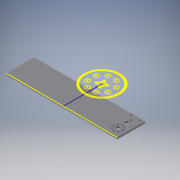
# Autodesk Inventor part: Winch Upright
Saved by Autodesk Inventor 2016 (Build 200138000, 138)
## iProperties
Created: 2015-12-16
Part Number: Winch Upright
Material: Generic
Document SubType Name: Modeling
Designer: Julia
Density: 1 g/cm^3
Appearance: Default
Author: Julia
Autodesk Inventor part; units mm, degrees
ref_plane "YZ Plane" through (0, 0, 0) normal (1, 0, 0) x (0, 1, 0)
ref_plane "XZ Plane" through (0, 0, 0) normal (0, 1, 0) x (-1, 0, 0)
ref_plane "XY Plane" through (0, 0, 0) normal (0, 0, 1) x (1, 0, 0)
sketch "Sketch1" plane through (0, 0, 0) normal (0, 1, 0) x (-1, 0, 0)
  line L0 (0, 0) -> (0, -50.8)
  line L1 (0, -50.8) -> (203.2, -50.8)
  line L2 (203.2, -50.8) -> (203.2, 0)
  line L3 (203.2, 0) -> (0, 0)
  dimension "d0" = 50.8
  dimension "d1" = 203.2
  constraints: 8 end point, 2 perpendicular, 1 horizontal, 1 vertical
  measures "d0" distance of L0.start L0.end
  measures "d1" distance of L0.end L1.end
extrude "Extrusion1" add sketch "Sketch1" along normal blind 3.302
sketch "Sketch2" plane through (0, 0, 0) normal (0, -1, 0) x (1, 0, 0)
  line L0 (-0.5, 0) -> (-0.5, -416) projected
  line L1 (-27.5, -416) -> (-0.5, -416) projected
  arc A0 (-30, -413.5) -> (-27.5, -416) centre (-27.5, -413.5) ccw projected
  line L2 (-30, -413.5) -> (-30, -2.5) projected
  arc A1 (-27.5, 0) -> (-30, -2.5) centre (-27.5, -2.5) ccw projected
  line L3 (-27.5, 0) -> (-0.5, 0) projected
  circle A2 centre (-14, -288) radius 4 projected
  circle A3 centre (-14, -320) radius 4 projected
  circle A4 centre (-14, -352) radius 4 projected
  circle A5 centre (-14, -384) radius 4 projected
  circle A6 centre (-14, -16) radius 4 projected
  circle A7 centre (-22, -16) radius 1.85 projected
  circle A8 centre (-6, -16) radius 1.85 projected
  circle A9 centre (-14, -24) radius 1.85 projected
  circle A10 centre (-14, -8) radius 1.85 projected
  circle A11 centre (-19.6569, -21.6569) radius 1.85 projected
  circle A12 centre (-19.6569, -10.3431) radius 1.85 projected
  circle A13 centre (-8.3431, -10.3431) radius 1.85 projected
  circle A14 centre (-8.3431, -21.6569) radius 1.85 projected
  circle A15 centre (-14, -80) radius 4 projected
  circle A16 centre (-22, -80) radius 1.85 projected
  circle A17 centre (-6, -80) radius 1.85 projected
  circle A18 centre (-14, -88) radius 1.85 projected
  circle A19 centre (-14, -72) radius 1.85 projected
  circle A20 centre (-19.6569, -85.6569) radius 1.85 projected
  circle A21 centre (-19.6569, -74.3431) radius 1.85 projected
  circle A22 centre (-8.3431, -74.3431) radius 1.85 projected
  circle A23 centre (-8.3431, -85.6569) radius 1.85 projected
  circle A24 centre (-14, -144) radius 4 projected
  circle A25 centre (-22, -144) radius 1.85 projected
  circle A26 centre (-6, -144) radius 1.85 projected
  circle A27 centre (-14, -152) radius 1.85 projected
  circle A28 centre (-14, -136) radius 1.85 projected
  circle A29 centre (-19.6569, -149.6569) radius 1.85 projected
  circle A30 centre (-19.6569, -138.3431) radius 1.85 projected
  circle A31 centre (-8.3431, -138.3431) radius 1.85 projected
  circle A32 centre (-8.3431, -149.6569) radius 1.85 projected
  circle A33 centre (-14, -208) radius 4 projected
  circle A34 centre (-22, -208) radius 1.85 projected
  circle A35 centre (-6, -208) radius 1.85 projected
  circle A36 centre (-14, -216) radius 1.85 projected
  circle A37 centre (-14, -200) radius 1.85 projected
  circle A38 centre (-19.6569, -213.6569) radius 1.85 projected
  circle A39 centre (-19.6569, -202.3431) radius 1.85 projected
  circle A40 centre (-8.3431, -202.3431) radius 1.85 projected
  circle A41 centre (-8.3431, -213.6569) radius 1.85 projected
  circle A42 centre (-14, -272) radius 4 projected
  circle A43 centre (-22, -272) radius 1.85 projected
  circle A44 centre (-6, -272) radius 1.85 projected
  circle A45 centre (-14, -280) radius 1.85 projected
  circle A46 centre (-14, -264) radius 1.85 projected
  circle A47 centre (-19.6569, -277.6569) radius 1.85 projected
  circle A48 centre (-19.6569, -266.3431) radius 1.85 projected
  circle A49 centre (-8.3431, -266.3431) radius 1.85 projected
  circle A50 centre (-8.3431, -277.6569) radius 1.85 projected
  circle A51 centre (-14, -336) radius 4 projected
  circle A52 centre (-22, -336) radius 1.85 projected
  circle A53 centre (-6, -336) radius 1.85 projected
  circle A54 centre (-14, -344) radius 1.85 projected
  circle A55 centre (-14, -328) radius 1.85 projected
  circle A56 centre (-19.6569, -341.6569) radius 1.85 projected
  circle A57 centre (-19.6569, -330.3431) radius 1.85 projected
  circle A58 centre (-8.3431, -330.3431) radius 1.85 projected
  circle A59 centre (-8.3431, -341.6569) radius 1.85 projected
  circle A60 centre (-14, -400) radius 4 projected
  circle A61 centre (-22, -400) radius 1.85 projected
  circle A62 centre (-6, -400) radius 1.85 projected
  circle A63 centre (-14, -408) radius 1.85 projected
  circle A64 centre (-14, -392) radius 1.85 projected
  circle A65 centre (-19.6569, -405.6569) radius 1.85 projected
  circle A66 centre (-19.6569, -394.3431) radius 1.85 projected
  circle A67 centre (-8.3431, -394.3431) radius 1.85 projected
  circle A68 centre (-8.3431, -405.6569) radius 1.85 projected
  circle A69 centre (-14, -48) radius 4 projected
  circle A70 centre (-22, -48) radius 1.85 projected
  circle A71 centre (-14, -56) radius 1.85 projected
  circle A72 centre (-6, -48) radius 1.85 projected
  circle A73 centre (-14, -40) radius 1.85 projected
  circle A74 centre (-14, -112) radius 4 projected
  circle A75 centre (-22, -112) radius 1.85 projected
  circle A76 centre (-14, -120) radius 1.85 projected
  circle A77 centre (-6, -112) radius 1.85 projected
  circle A78 centre (-14, -104) radius 1.85 projected
  circle A79 centre (-14, -176) radius 4 projected
  circle A80 centre (-22, -176) radius 1.85 projected
  circle A81 centre (-14, -184) radius 1.85 projected
  circle A82 centre (-6, -176) radius 1.85 projected
  circle A83 centre (-14, -168) radius 1.85 projected
  circle A84 centre (-14, -240) radius 4 projected
  circle A85 centre (-22, -240) radius 1.85 projected
  circle A86 centre (-14, -248) radius 1.85 projected
  circle A87 centre (-6, -240) radius 1.85 projected
  circle A88 centre (-14, -232) radius 1.85 projected
  circle A89 centre (-14, -304) radius 4 projected
  circle A90 centre (-22, -304) radius 1.85 projected
  circle A91 centre (-14, -312) radius 1.85 projected
  circle A92 centre (-6, -304) radius 1.85 projected
  circle A93 centre (-14, -296) radius 1.85 projected
  circle A94 centre (-14, -368) radius 4 projected
  circle A95 centre (-22, -368) radius 1.85 projected
  circle A96 centre (-14, -376) radius 1.85 projected
  circle A97 centre (-6, -368) radius 1.85 projected
  circle A98 centre (-14, -360) radius 1.85 projected
  circle A99 centre (-14, -32) radius 4 projected
  circle A100 centre (-14, -64) radius 4 projected
  circle A101 centre (-14, -96) radius 4 projected
  circle A102 centre (-14, -128) radius 4 projected
  circle A103 centre (-14, -160) radius 4 projected
  circle A104 centre (-14, -192) radius 4 projected
  circle A105 centre (-14, -224) radius 4 projected
  circle A106 centre (-14, -256) radius 4 projected
  point P0 (0, 0)
extrude "Extrusion2" cut sketch "Sketch2" against normal blind 20.5105 contours A6 | A7 | A8 | A9 | A10 | A11 | A12 | A13 | A14 | A70 | A72 | A73 | A99
sketch "Sketch3" plane through (0, 3.302, 0) normal (0, 1, 0) x (1, 0, 0)
  circle A0 centre (-98.9805, 70.6479) radius 6 projected
  arc A1 (-126.4697, 56.3203) -> (-127.7519, 54.8984) centre (-117.6318, 47.0611) ccw projected
  arc A2 (-127.7519, 54.8984) -> (-127.494, 54.4363) centre (-98.9805, 70.6479) ccw projected
  arc A3 (-127.494, 54.4363) -> (-125.6107, 54.7807) centre (-128.8482, 67.1645) ccw projected
  arc A4 (-125.6107, 54.7807) -> (-125.2608, 54.2076) centre (-98.9805, 70.6479) ccw projected
  arc A5 (-125.2608, 54.2076) -> (-126.4275, 52.6896) centre (-115.7237, 45.6704) ccw projected
  arc A6 (-126.4275, 52.6896) -> (-126.1342, 52.2491) centre (-98.9805, 70.6479) ccw projected
  arc A7 (-126.1342, 52.2491) -> (-124.2837, 52.7402) centre (-128.4828, 64.8318) ccw projected
  arc A8 (-124.2837, 52.7402) -> (-123.8899, 52.1964) centre (-98.9805, 70.6479) ccw projected
  arc A9 (-123.8899, 52.1964) -> (-124.9339, 50.5915) centre (-113.7124, 44.4337) ccw projected
  arc A10 (-124.9339, 50.5915) -> (-124.6069, 50.1754) centre (-98.9805, 70.6479) ccw projected
  arc A11 (-124.6069, 50.1754) -> (-122.8006, 50.8101) centre (-127.9355, 62.535) ccw projected
  arc A12 (-122.8006, 50.8101) -> (-122.3654, 50.2989) centre (-98.9805, 70.6479) ccw projected
  arc A13 (-122.3654, 50.2989) -> (-123.2803, 48.6171) centre (-111.6103, 43.3587) ccw projected
  arc A14 (-123.2803, 48.6171) -> (-122.9217, 48.2279) centre (-98.9805, 70.6479) ccw projected
  arc A15 (-122.9217, 48.2279) -> (-121.1708, 49.0024) centre (-127.2098, 60.2882) ccw projected
  arc A16 (-121.1708, 49.0024) -> (-120.6968, 48.5269) centre (-98.9805, 70.6479) ccw projected
  arc A17 (-120.6968, 48.5269) -> (-121.4768, 46.7784) centre (-109.4302, 42.4519) ccw projected
  arc A18 (-121.4768, 46.7784) -> (-121.0888, 46.4186) centre (-98.9805, 70.6479) ccw projected
  arc A19 (-121.0888, 46.4186) -> (-119.4041, 47.3281) centre (-126.3099, 58.1053) ccw projected
  arc A20 (-119.4041, 47.3281) -> (-118.8942, 46.8912) centre (-98.9805, 70.6479) ccw projected
  arc A21 (-118.8942, 46.8912) -> (-119.5347, 45.087) centre (-107.1858, 41.7189) ccw projected
  arc A22 (-119.5347, 45.087) -> (-119.1197, 44.7587) centre (-98.9805, 70.6479) ccw projected
  arc A23 (-119.1197, 44.7587) -> (-117.5114, 45.7976) centre (-125.2416, 55.9998) ccw projected
  arc A24 (-117.5114, 45.7976) -> (-116.9689, 45.4021) centre (-98.9805, 70.6479) ccw projected
  arc A25 (-116.9689, 45.4021) -> (-117.4659, 43.5531) centre (-104.8907, 41.1643) ccw projected
  arc A26 (-117.4659, 43.5531) -> (-117.0263, 43.2584) centre (-98.9805, 70.6479) ccw projected
  arc A27 (-117.0263, 43.2584) -> (-115.5046, 44.4202) centre (-124.0114, 53.9845) ccw projected
  arc A28 (-115.5046, 44.4202) -> (-114.9327, 44.0685) centre (-98.9805, 70.6479) ccw projected
  arc A29 (-114.9327, 44.0685) -> (-115.283, 42.1863) centre (-102.5593, 40.7915) ccw projected
  arc A30 (-115.283, 42.1863) -> (-114.8217, 41.927) centre (-98.9805, 70.6479) ccw projected
  arc A31 (-114.8217, 41.927) -> (-113.3958, 43.2046) centre (-122.6268, 52.072) ccw projected
  arc A32 (-113.3958, 43.2046) -> (-112.7981, 42.8989) centre (-98.9805, 70.6479) ccw projected
  arc A33 (-112.7981, 42.8989) -> (-112.9997, 40.9949) centre (-100.2057, 40.6028) ccw projected
  arc A34 (-112.9997, 40.9949) -> (-112.5195, 40.7726) centre (-98.9805, 70.6479) ccw projected
  arc A35 (-112.5195, 40.7726) -> (-111.1982, 42.1582) centre (-121.0964, 50.274) ccw projected
  arc A36 (-111.1982, 42.1582) -> (-110.5783, 41.9003) centre (-98.9805, 70.6479) ccw projected
  arc A37 (-110.5783, 41.9003) -> (-110.6299, 39.9864) centre (-97.8446, 40.5992) ccw projected
  arc A38 (-110.6299, 39.9864) -> (-110.1337, 39.8024) centre (-98.9805, 70.6479) ccw projected
  arc A39 (-110.1337, 39.8024) -> (-108.9253, 41.2874) centre (-119.4297, 48.6016) ccw projected
  arc A40 (-108.9253, 41.2874) -> (-108.2871, 41.0789) centre (-98.9805, 70.6479) ccw projected
  arc A41 (-108.2871, 41.0789) -> (-108.1884, 39.1669) centre (-95.4905, 40.781) ccw projected
  arc A42 (-108.1884, 39.1669) -> (-107.6793, 39.0225) centre (-98.9805, 70.6479) ccw projected
  arc A43 (-107.6793, 39.0225) -> (-106.591, 40.5977) centre (-117.637, 47.0651) ccw projected
  arc A44 (-106.591, 40.5977) -> (-105.9384, 40.4399) centre (-98.9805, 70.6479) ccw projected
  arc A45 (-105.9384, 40.4399) -> (-105.69, 38.5415) centre (-93.158, 41.1469) ccw projected
  arc A46 (-105.69, 38.5415) -> (-105.1711, 38.4375) centre (-98.9805, 70.6479) ccw projected
  arc A47 (-105.1711, 38.4375) -> (-104.2099, 40.0932) centre (-115.7292, 45.674) ccw projected
  arc A48 (-104.2099, 40.0932) -> (-103.5469, 39.9871) centre (-98.9805, 70.6479) ccw projected
  arc A49 (-103.5469, 39.9871) -> (-103.1503, 38.1141) centre (-90.8613, 41.6947) ccw projected
  arc A50 (-103.1503, 38.1141) -> (-102.6248, 38.051) centre (-98.9805, 70.6479) ccw projected
  arc A51 (-102.6248, 38.051) -> (-101.7964, 39.7771) centre (-113.7181, 44.4369) ccw projected
  arc A52 (-101.7964, 39.7771) -> (-101.1272, 39.7234) centre (-98.9805, 70.6479) ccw projected
  arc A53 (-101.1272, 39.7234) -> (-100.5848, 37.8872) centre (-88.6147, 42.4209) ccw projected
  arc A54 (-100.5848, 37.8872) -> (-100.0561, 37.8656) centre (-98.9805, 70.6479) ccw projected
  arc A55 (-100.0561, 37.8656) -> (-99.3657, 39.6513) centre (-111.6162, 43.3614) ccw projected
  arc A56 (-99.3657, 39.6513) -> (-98.6942, 39.6503) centre (-98.9805, 70.6479) ccw projected
  arc A57 (-98.6942, 39.6503) -> (-98.0095, 37.8623) centre (-86.4319, 43.3212) ccw projected
  arc A58 (-98.0095, 37.8623) -> (-97.4807, 37.8823) centre (-98.9805, 70.6479) ccw projected
  arc A59 (-97.4807, 37.8823) -> (-96.9325, 39.7167) centre (-109.4364, 42.4542) ccw projected
  arc A60 (-96.9325, 39.7167) -> (-96.2631, 39.7683) centre (-98.9805, 70.6479) ccw projected
  arc A61 (-96.2631, 39.7683) -> (-95.4402, 38.0396) centre (-84.3266, 44.39) ccw projected
  arc A62 (-95.4402, 38.0396) -> (-94.9146, 38.1009) centre (-98.9805, 70.6479) ccw projected
  arc A63 (-94.9146, 38.1009) -> (-94.512, 39.9727) centre (-107.1921, 41.7207) ccw projected
  arc A64 (-94.512, 39.9727) -> (-93.8487, 40.0767) centre (-98.9805, 70.6479) ccw projected
  arc A65 (-93.8487, 40.0767) -> (-92.8927, 38.4179) centre (-82.3116, 45.6207) ccw projected
  arc A66 (-92.8927, 38.4179) -> (-92.3735, 38.5203) centre (-98.9805, 70.6479) ccw projected
  arc A67 (-92.3735, 38.5203) -> (-92.119, 40.4179) centre (-104.8971, 41.1656) ccw projected
  arc A68 (-92.119, 40.4179) -> (-91.4659, 40.5736) centre (-98.9805, 70.6479) ccw projected
  arc A69 (-91.4659, 40.5736) -> (-90.3827, 38.9949) centre (-80.3994, 47.0057) ccw projected
  arc A70 (-90.3827, 38.9949) -> (-89.8731, 39.1377) centre (-98.9805, 70.6479) ccw projected
  arc A71 (-89.8731, 39.1377) -> (-89.7683, 41.0494) centre (-102.5657, 40.7923) ccw projected
  arc A72 (-89.7683, 41.0494) -> (-89.1294, 41.2559) centre (-98.9805, 70.6479) ccw projected
  arc A73 (-89.1294, 41.2559) -> (-87.9257, 39.767) centre (-78.6017, 48.5364) ccw projected
  arc A74 (-87.9257, 39.767) -> (-87.4289, 39.9494) centre (-98.9805, 70.6479) ccw projected
  arc A75 (-87.4289, 39.9494) -> (-87.4745, 41.8634) centre (-100.2122, 40.603) ccw projected
  arc A76 (-87.4745, 41.8634) -> (-86.8537, 42.1194) centre (-98.9805, 70.6479) ccw projected
  arc A77 (-86.8537, 42.1194) -> (-85.5369, 40.7296) centre (-76.9297, 50.2035) ccw projected
  arc A78 (-85.5369, 40.7296) -> (-85.056, 40.9503) centre (-98.9805, 70.6479) ccw projected
  arc A79 (-85.056, 40.9503) -> (-85.2515, 42.8549) centre (-97.8512, 40.599) ccw projected
  arc A80 (-85.2515, 42.8549) -> (-84.6528, 43.1588) centre (-98.9805, 70.6479) ccw projected
  arc A81 (-84.6528, 43.1588) -> (-83.231, 41.8765) centre (-75.3936, 51.9966) ccw projected
  arc A82 (-83.231, 41.8765) -> (-82.7689, 42.1344) centre (-98.9805, 70.6479) ccw projected
  arc A83 (-82.7689, 42.1344) -> (-83.1132, 44.0177) centre (-95.497, 40.7802) ccw projected
  arc A84 (-83.1132, 44.0177) -> (-82.5402, 44.3676) centre (-98.9805, 70.6479) ccw projected
  arc A85 (-82.5402, 44.3676) -> (-81.0222, 43.2009) centre (-74.0029, 53.9047) ccw projected
  arc A86 (-81.0222, 43.2009) -> (-80.5817, 43.4942) centre (-98.9805, 70.6479) ccw projected
  arc A87 (-80.5817, 43.4942) -> (-81.0727, 45.3448) centre (-93.1644, 41.1456) ccw projected
  arc A88 (-81.0727, 45.3448) -> (-80.5289, 45.7385) centre (-98.9805, 70.6479) ccw projected
  arc A89 (-80.5289, 45.7385) -> (-78.9241, 44.6945) centre (-72.7663, 55.916) ccw projected
  arc A90 (-78.9241, 44.6945) -> (-78.5079, 45.0215) centre (-98.9805, 70.6479) ccw projected
  arc A91 (-78.5079, 45.0215) -> (-79.1427, 46.8278) centre (-90.8676, 41.6929) ccw projected
  arc A92 (-79.1427, 46.8278) -> (-78.6314, 47.263) centre (-98.9805, 70.6479) ccw projected
  arc A93 (-78.6314, 47.263) -> (-76.9496, 46.3482) centre (-71.6912, 58.0182) ccw projected
  arc A94 (-76.9496, 46.3482) -> (-76.5604, 46.7068) centre (-98.9805, 70.6479) ccw projected
  arc A95 (-76.5604, 46.7068) -> (-77.3349, 48.4577) centre (-88.6208, 42.4187) ccw projected
  arc A96 (-77.3349, 48.4577) -> (-76.8594, 48.9317) centre (-98.9805, 70.6479) ccw projected
  arc A97 (-76.8594, 48.9317) -> (-75.111, 48.1516) centre (-70.7844, 60.1982) ccw projected
  arc A98 (-75.111, 48.1516) -> (-74.7511, 48.5396) centre (-98.9805, 70.6479) ccw projected
  arc A99 (-74.7511, 48.5396) -> (-75.6606, 50.2244) centre (-86.4379, 43.3185) ccw projected
  arc A100 (-75.6606, 50.2244) -> (-75.2238, 50.7342) centre (-98.9805, 70.6479) ccw projected
  arc A101 (-75.2238, 50.7342) -> (-73.4195, 50.0937) centre (-70.0515, 62.4427) ccw projected
  arc A102 (-73.4195, 50.0937) -> (-73.0912, 50.5088) centre (-98.9805, 70.6479) ccw projected
  arc A103 (-73.0912, 50.5088) -> (-74.1301, 52.117) centre (-84.3323, 44.3868) ccw projected
  arc A104 (-74.1301, 52.117) -> (-73.7346, 52.6595) centre (-98.9805, 70.6479) ccw projected
  arc A105 (-73.7346, 52.6595) -> (-71.8856, 52.1626) centre (-69.4969, 64.7377) ccw projected
  arc A106 (-71.8856, 52.1626) -> (-71.5909, 52.6021) centre (-98.9805, 70.6479) ccw projected
  arc A107 (-71.5909, 52.6021) -> (-72.7528, 54.1239) centre (-82.317, 45.6171) ccw projected
  arc A108 (-72.7528, 54.1239) -> (-72.4011, 54.6958) centre (-98.9805, 70.6479) ccw projected
  arc A109 (-72.4011, 54.6958) -> (-70.5188, 54.3454) centre (-69.124, 67.0692) ccw projected
  arc A110 (-70.5188, 54.3454) -> (-70.2595, 54.8067) centre (-98.9805, 70.6479) ccw projected
  arc A111 (-70.2595, 54.8067) -> (-71.5372, 56.2326) centre (-80.4045, 47.0016) ccw projected
  arc A112 (-71.5372, 56.2326) -> (-71.2314, 56.8303) centre (-98.9805, 70.6479) ccw projected
  arc A113 (-71.2314, 56.8303) -> (-69.3275, 56.6287) centre (-68.9353, 69.4227) ccw projected
  arc A114 (-69.3275, 56.6287) -> (-69.1051, 57.109) centre (-98.9805, 70.6479) ccw projected
  arc A115 (-69.1051, 57.109) -> (-70.4908, 58.4302) centre (-78.6065, 48.532) ccw projected
  arc A116 (-70.4908, 58.4302) -> (-70.2328, 59.0501) centre (-98.9805, 70.6479) ccw projected
  arc A117 (-70.2328, 59.0501) -> (-68.3189, 58.9985) centre (-68.9318, 71.7838) ccw projected
  arc A118 (-68.3189, 58.9985) -> (-68.135, 59.4947) centre (-98.9805, 70.6479) ccw projected
  arc A119 (-68.135, 59.4947) -> (-69.62, 60.7031) centre (-76.9341, 50.1987) ccw projected
  arc A120 (-69.62, 60.7031) -> (-69.4115, 61.3414) centre (-98.9805, 70.6479) ccw projected
  arc A121 (-69.4115, 61.3414) -> (-67.4995, 61.4401) centre (-69.1135, 74.1379) ccw projected
  arc A122 (-67.4995, 61.4401) -> (-67.355, 61.9492) centre (-98.9805, 70.6479) ccw projected
  arc A123 (-67.355, 61.9492) -> (-68.9302, 63.0374) centre (-75.3976, 51.9915) ccw projected
  arc A124 (-68.9302, 63.0374) -> (-68.7725, 63.69) centre (-98.9805, 70.6479) ccw projected
  arc A125 (-68.7725, 63.69) -> (-66.8741, 63.9384) centre (-69.4794, 76.4705) ccw projected
  arc A126 (-66.8741, 63.9384) -> (-66.77, 64.4573) centre (-98.9805, 70.6479) ccw projected
  arc A127 (-66.77, 64.4573) -> (-68.4258, 65.4186) centre (-74.0066, 53.8993) ccw projected
  arc A128 (-68.4258, 65.4186) -> (-68.3197, 66.0816) centre (-98.9805, 70.6479) ccw projected
  arc A129 (-68.3197, 66.0816) -> (-66.4466, 66.4782) centre (-70.0272, 78.7672) ccw projected
  arc A130 (-66.4466, 66.4782) -> (-66.3836, 67.0036) centre (-98.9805, 70.6479) ccw projected
  arc A131 (-66.3836, 67.0036) -> (-68.1097, 67.832) centre (-72.7695, 55.9103) ccw projected
  arc A132 (-68.1097, 67.832) -> (-68.0559, 68.5013) centre (-98.9805, 70.6479) ccw projected
  arc A133 (-68.0559, 68.5013) -> (-66.2197, 69.0436) centre (-70.7535, 81.0138) ccw projected
  arc A134 (-66.2197, 69.0436) -> (-66.1981, 69.5723) centre (-98.9805, 70.6479) ccw projected
  arc A135 (-66.1981, 69.5723) -> (-67.9839, 70.2628) centre (-71.694, 58.0123) ccw projected
  arc A136 (-67.9839, 70.2628) -> (-67.9828, 70.9342) centre (-98.9805, 70.6479) ccw projected
  arc A137 (-67.9828, 70.9342) -> (-66.1949, 71.6189) centre (-71.6538, 83.1965) ccw projected
  arc A138 (-66.1949, 71.6189) -> (-66.2148, 72.1477) centre (-98.9805, 70.6479) ccw projected
  arc A139 (-66.2148, 72.1477) -> (-68.0492, 72.6959) centre (-70.7867, 60.1921) ccw projected
  arc A140 (-68.0492, 72.6959) -> (-68.1008, 73.3654) centre (-98.9805, 70.6479) ccw projected
  arc A141 (-68.1008, 73.3654) -> (-66.3721, 74.1882) centre (-72.7226, 85.3018) ccw projected
  arc A142 (-66.3721, 74.1882) -> (-66.4335, 74.7139) centre (-98.9805, 70.6479) ccw projected
  arc A143 (-66.4335, 74.7139) -> (-68.3052, 75.1165) centre (-70.0533, 62.4364) ccw projected
  arc A144 (-68.3052, 75.1165) -> (-68.4092, 75.7798) centre (-98.9805, 70.6479) ccw projected
  arc A145 (-68.4092, 75.7798) -> (-66.7504, 76.7358) centre (-73.9532, 87.3168) ccw projected
  arc A146 (-66.7504, 76.7358) -> (-66.8528, 77.255) centre (-98.9805, 70.6479) ccw projected
  arc A147 (-66.8528, 77.255) -> (-68.7504, 77.5094) centre (-69.4982, 64.7313) ccw projected
  arc A148 (-68.7504, 77.5094) -> (-68.9061, 78.1625) centre (-98.9805, 70.6479) ccw projected
  arc A149 (-68.9061, 78.1625) -> (-67.3274, 79.2457) centre (-75.3382, 89.2291) ccw projected
  arc A150 (-67.3274, 79.2457) -> (-67.4702, 79.7553) centre (-98.9805, 70.6479) ccw projected
  arc A151 (-67.4702, 79.7553) -> (-69.3819, 79.8601) centre (-69.1248, 67.0627) ccw projected
  arc A152 (-69.3819, 79.8601) -> (-69.5884, 80.499) centre (-98.9805, 70.6479) ccw projected
  arc A153 (-69.5884, 80.499) -> (-68.0995, 81.7027) centre (-76.869, 91.0267) ccw projected
  arc A154 (-68.0995, 81.7027) -> (-68.2819, 82.1995) centre (-98.9805, 70.6479) ccw projected
  arc A155 (-68.2819, 82.1995) -> (-70.196, 82.154) centre (-68.9356, 69.4162) ccw projected
  arc A156 (-70.196, 82.154) -> (-70.4519, 82.7747) centre (-98.9805, 70.6479) ccw projected
  arc A157 (-70.4519, 82.7747) -> (-69.0621, 84.0915) centre (-78.536, 92.6988) ccw projected
  arc A158 (-69.0621, 84.0915) -> (-69.2829, 84.5725) centre (-98.9805, 70.6479) ccw projected
  arc A159 (-69.2829, 84.5725) -> (-71.1874, 84.3769) centre (-68.9315, 71.7773) ccw projected
  arc A160 (-71.1874, 84.3769) -> (-71.4913, 84.9756) centre (-98.9805, 70.6479) ccw projected
  arc A161 (-71.4913, 84.9756) -> (-70.2091, 86.3974) centre (-80.3291, 94.2348) ccw projected
  arc A162 (-70.2091, 86.3974) -> (-70.4669, 86.8596) centre (-98.9805, 70.6479) ccw projected
  arc A163 (-70.4669, 86.8596) -> (-72.3503, 86.5152) centre (-69.1128, 74.1314) ccw projected
  arc A164 (-72.3503, 86.5152) -> (-72.7002, 87.0882) centre (-98.9805, 70.6479) ccw projected
  arc A165 (-72.7002, 87.0882) -> (-71.5335, 88.6063) centre (-82.2372, 95.6255) ccw projected
  arc A166 (-71.5335, 88.6063) -> (-71.8268, 89.0468) centre (-98.9805, 70.6479) ccw projected
  arc A167 (-71.8268, 89.0468) -> (-73.6773, 88.5557) centre (-69.4782, 76.4641) ccw projected
  arc A168 (-73.6773, 88.5557) -> (-74.0711, 89.0995) centre (-98.9805, 70.6479) ccw projected
  arc A169 (-74.0711, 89.0995) -> (-73.0271, 90.7044) centre (-84.2486, 96.8622) ccw projected
  arc A170 (-73.0271, 90.7044) -> (-73.354, 91.1205) centre (-98.9805, 70.6479) ccw projected
  arc A171 (-73.354, 91.1205) -> (-75.1603, 90.4857) centre (-70.0254, 78.7609) ccw projected
  arc A172 (-75.1603, 90.4857) -> (-75.5956, 90.997) centre (-98.9805, 70.6479) ccw projected
  arc A173 (-75.5956, 90.997) -> (-74.6807, 92.6788) centre (-86.3507, 97.9372) ccw projected
  arc A174 (-74.6807, 92.6788) -> (-75.0393, 93.068) centre (-98.9805, 70.6479) ccw projected
  arc A175 (-75.0393, 93.068) -> (-76.7902, 92.2935) centre (-70.7512, 81.0076) ccw projected
  arc A176 (-76.7902, 92.2935) -> (-77.2642, 92.769) centre (-98.9805, 70.6479) ccw projected
  arc A177 (-77.2642, 92.769) -> (-76.4841, 94.5175) centre (-88.5307, 98.844) ccw projected
  arc A178 (-76.4841, 94.5175) -> (-76.8722, 94.8773) centre (-98.9805, 70.6479) ccw projected
  arc A179 (-76.8722, 94.8773) -> (-78.5569, 93.9678) centre (-71.6511, 83.1906) ccw projected
  arc A180 (-78.5569, 93.9678) -> (-79.0668, 94.4047) centre (-98.9805, 70.6479) ccw projected
  arc A181 (-79.0668, 94.4047) -> (-78.4263, 96.2089) centre (-90.7752, 99.577) ccw projected
  arc A182 (-78.4263, 96.2089) -> (-78.8413, 96.5372) centre (-98.9805, 70.6479) ccw projected
  arc A183 (-78.8413, 96.5372) -> (-80.4495, 95.4983) centre (-72.7194, 85.2961) ccw projected
  arc A184 (-80.4495, 95.4983) -> (-80.9921, 95.8938) centre (-98.9805, 70.6479) ccw projected
  arc A185 (-80.9921, 95.8938) -> (-80.4951, 97.7428) centre (-93.0702, 100.1316) ccw projected
  arc A186 (-80.4951, 97.7428) -> (-80.9347, 98.0375) centre (-98.9805, 70.6479) ccw projected
  arc A187 (-80.9347, 98.0375) -> (-82.4564, 96.8756) centre (-73.9496, 87.3114) ccw projected
  arc A188 (-82.4564, 96.8756) -> (-83.0283, 97.2274) centre (-98.9805, 70.6479) ccw projected
  arc A189 (-83.0283, 97.2274) -> (-82.6779, 99.1096) centre (-95.4017, 100.5044) ccw projected
  arc A190 (-82.6779, 99.1096) -> (-83.1392, 99.3689) centre (-98.9805, 70.6479) ccw projected
  arc A191 (-83.1392, 99.3689) -> (-84.5651, 98.0913) centre (-75.3342, 89.2239) ccw projected
  arc A192 (-84.5651, 98.0913) -> (-85.1629, 98.397) centre (-98.9805, 70.6479) ccw projected
  arc A193 (-85.1629, 98.397) -> (-84.9613, 100.301) centre (-97.7552, 100.6931) ccw projected
  arc A194 (-84.9613, 100.301) -> (-85.4415, 100.5233) centre (-98.9805, 70.6479) ccw projected
  arc A195 (-85.4415, 100.5233) -> (-86.7627, 99.1377) centre (-76.8645, 91.0219) ccw projected
  arc A196 (-86.7627, 99.1377) -> (-87.3826, 99.3956) centre (-98.9805, 70.6479) ccw projected
  arc A197 (-87.3826, 99.3956) -> (-87.331, 101.3095) centre (-100.1163, 100.6966) ccw projected
  arc A198 (-87.331, 101.3095) -> (-87.8272, 101.4934) centre (-98.9805, 70.6479) ccw projected
  arc A199 (-87.8272, 101.4934) -> (-89.0357, 100.0084) centre (-78.5312, 92.6943) ccw projected
  arc A200 (-89.0357, 100.0084) -> (-89.6739, 100.2169) centre (-98.9805, 70.6479) ccw projected
  arc A201 (-89.6739, 100.2169) -> (-89.7726, 102.129) centre (-102.4704, 100.5149) ccw projected
  arc A202 (-89.7726, 102.129) -> (-90.2817, 102.2734) centre (-98.9805, 70.6479) ccw projected
  arc A203 (-90.2817, 102.2734) -> (-91.3699, 100.6982) centre (-80.324, 94.2308) ccw projected
  arc A204 (-91.3699, 100.6982) -> (-92.0226, 100.856) centre (-98.9805, 70.6479) ccw projected
  arc A205 (-92.0226, 100.856) -> (-92.271, 102.7544) centre (-104.803, 100.149) ccw projected
  arc A206 (-92.271, 102.7544) -> (-92.7898, 102.8584) centre (-98.9805, 70.6479) ccw projected
  arc A207 (-92.7898, 102.8584) -> (-93.7511, 101.2027) centre (-82.2318, 95.6219) ccw projected
  arc A208 (-93.7511, 101.2027) -> (-94.4141, 101.3088) centre (-98.9805, 70.6479) ccw projected
  arc A209 (-94.4141, 101.3088) -> (-94.8107, 103.1818) centre (-107.0997, 99.6012) ccw projected
  arc A210 (-94.8107, 103.1818) -> (-95.3361, 103.2449) centre (-98.9805, 70.6479) ccw projected
  arc A211 (-95.3361, 103.2449) -> (-96.1645, 101.5188) centre (-84.2429, 96.859) ccw projected
  arc A212 (-96.1645, 101.5188) -> (-96.8338, 101.5725) centre (-98.9805, 70.6479) ccw projected
  arc A213 (-96.8338, 101.5725) -> (-97.3761, 103.4087) centre (-109.3463, 98.875) ccw projected
  arc A214 (-97.3761, 103.4087) -> (-97.9049, 103.4303) centre (-98.9805, 70.6479) ccw projected
  arc A215 (-97.9049, 103.4303) -> (-98.5953, 101.6446) centre (-86.3448, 97.9345) ccw projected
  arc A216 (-98.5953, 101.6446) -> (-99.2667, 101.6456) centre (-98.9805, 70.6479) ccw projected
  arc A217 (-99.2667, 101.6456) -> (-99.9514, 103.4336) centre (-111.529, 97.9747) ccw projected
  arc A218 (-99.9514, 103.4336) -> (-100.4803, 103.4136) centre (-98.9805, 70.6479) ccw projected
  arc A219 (-100.4803, 103.4136) -> (-101.0285, 101.5792) centre (-88.5246, 98.8417) ccw projected
  arc A220 (-101.0285, 101.5792) -> (-101.6979, 101.5276) centre (-98.9805, 70.6479) ccw projected
  arc A221 (-101.6979, 101.5276) -> (-102.5208, 103.2563) centre (-113.6344, 96.9059) ccw projected
  arc A222 (-102.5208, 103.2563) -> (-103.0464, 103.195) centre (-98.9805, 70.6479) ccw projected
  arc A223 (-103.0464, 103.195) -> (-103.449, 101.3232) centre (-90.7689, 99.5752) ccw projected
  arc A224 (-103.449, 101.3232) -> (-104.1123, 101.2192) centre (-98.9805, 70.6479) ccw projected
  arc A225 (-104.1123, 101.2192) -> (-105.0683, 102.878) centre (-115.6494, 95.6752) ccw projected
  arc A226 (-105.0683, 102.878) -> (-105.5875, 102.7756) centre (-98.9805, 70.6479) ccw projected
  arc A227 (-105.5875, 102.7756) -> (-105.842, 100.878) centre (-93.0638, 100.1303) ccw projected
  arc A228 (-105.842, 100.878) -> (-106.4951, 100.7223) centre (-98.9805, 70.6479) ccw projected
  arc A229 (-106.4951, 100.7223) -> (-107.5783, 102.301) centre (-117.5616, 94.2902) ccw projected
  arc A230 (-107.5783, 102.301) -> (-108.0878, 102.1582) centre (-98.9805, 70.6479) ccw projected
  arc A231 (-108.0878, 102.1582) -> (-108.1926, 100.2465) centre (-95.3952, 100.5036) ccw projected
  arc A232 (-108.1926, 100.2465) -> (-108.8315, 100.04) centre (-98.9805, 70.6479) ccw projected
  arc A233 (-108.8315, 100.04) -> (-110.0352, 101.5289) centre (-119.3593, 92.7595) ccw projected
  arc A234 (-110.0352, 101.5289) -> (-110.532, 101.3465) centre (-98.9805, 70.6479) ccw projected
  arc A235 (-110.532, 101.3465) -> (-110.4865, 99.4325) centre (-97.7487, 100.6929) ccw projected
  arc A236 (-110.4865, 99.4325) -> (-111.1072, 99.1765) centre (-98.9805, 70.6479) ccw projected
  arc A237 (-111.1072, 99.1765) -> (-112.4241, 100.5663) centre (-121.0313, 91.0924) ccw projected
  arc A238 (-112.4241, 100.5663) -> (-112.905, 100.3456) centre (-98.9805, 70.6479) ccw projected
  arc A239 (-112.905, 100.3456) -> (-112.7095, 98.441) centre (-100.1098, 100.6969) ccw projected
  arc A240 (-112.7095, 98.441) -> (-113.3082, 98.1371) centre (-98.9805, 70.6479) ccw projected
  arc A241 (-113.3082, 98.1371) -> (-114.73, 99.4193) centre (-122.5674, 89.2993) ccw projected
  arc A242 (-114.73, 99.4193) -> (-115.1921, 99.1615) centre (-98.9805, 70.6479) ccw projected
  arc A243 (-115.1921, 99.1615) -> (-114.8478, 97.2782) centre (-102.464, 100.5157) ccw projected
  arc A244 (-114.8478, 97.2782) -> (-115.4208, 96.9283) centre (-98.9805, 70.6479) ccw projected
  arc A245 (-115.4208, 96.9283) -> (-116.9388, 98.095) centre (-123.958, 87.3912) ccw projected
  arc A246 (-116.9388, 98.095) -> (-117.3793, 97.8017) centre (-98.9805, 70.6479) ccw projected
  arc A247 (-117.3793, 97.8017) -> (-116.8882, 95.9511) centre (-104.7966, 100.1503) ccw projected
  arc A248 (-116.8882, 95.9511) -> (-117.432, 95.5573) centre (-98.9805, 70.6479) ccw projected
  arc A249 (-117.432, 95.5573) -> (-119.0369, 96.6014) centre (-125.1947, 85.3799) ccw projected
  arc A250 (-119.0369, 96.6014) -> (-119.453, 96.2744) centre (-98.9805, 70.6479) ccw projected
  arc A251 (-119.453, 96.2744) -> (-118.8183, 94.4681) centre (-107.0934, 99.603) ccw projected
  arc A252 (-118.8183, 94.4681) -> (-119.3295, 94.0329) centre (-98.9805, 70.6479) ccw projected
  arc A253 (-119.3295, 94.0329) -> (-121.0114, 94.9477) centre (-126.2697, 83.2777) ccw projected
  arc A254 (-121.0114, 94.9477) -> (-121.4006, 94.5891) centre (-98.9805, 70.6479) ccw projected
  arc A255 (-121.4006, 94.5891) -> (-120.626, 92.8382) centre (-109.3402, 98.8772) ccw projected
  arc A256 (-120.626, 92.8382) -> (-121.1016, 92.3642) centre (-98.9805, 70.6479) ccw projected
  arc A257 (-121.1016, 92.3642) -> (-122.85, 93.1443) centre (-127.1765, 81.0977) ccw projected
  arc A258 (-122.85, 93.1443) -> (-123.2098, 92.7563) centre (-98.9805, 70.6479) ccw projected
  arc A259 (-123.2098, 92.7563) -> (-122.3003, 91.0715) centre (-111.5231, 97.9774) ccw projected
  arc A260 (-122.3003, 91.0715) -> (-122.7372, 90.5617) centre (-98.9805, 70.6479) ccw projected
  arc A261 (-122.7372, 90.5617) -> (-124.5415, 91.2022) centre (-127.9095, 78.8532) ccw projected
  arc A262 (-124.5415, 91.2022) -> (-124.8697, 90.7871) centre (-98.9805, 70.6479) ccw projected
  arc A263 (-124.8697, 90.7871) -> (-123.8309, 89.1789) centre (-113.6287, 96.909) ccw projected
  arc A264 (-123.8309, 89.1789) -> (-124.2264, 88.6364) centre (-98.9805, 70.6479) ccw projected
  arc A265 (-124.2264, 88.6364) -> (-126.0753, 89.1333) centre (-128.4641, 76.5582) ccw projected
  arc A266 (-126.0753, 89.1333) -> (-126.37, 88.6938) centre (-98.9805, 70.6479) ccw projected
  arc A267 (-126.37, 88.6938) -> (-125.2082, 87.172) centre (-115.6439, 95.6788) ccw projected
  arc A268 (-125.2082, 87.172) -> (-125.5599, 86.6001) centre (-98.9805, 70.6479) ccw projected
  arc A269 (-125.5599, 86.6001) -> (-127.4422, 86.9505) centre (-128.8369, 74.2267) ccw projected
  arc A270 (-127.4422, 86.9505) -> (-127.7015, 86.4892) centre (-98.9805, 70.6479) ccw projected
  arc A271 (-127.7015, 86.4892) -> (-126.4238, 85.0633) centre (-117.5565, 94.2943) ccw projected
  arc A272 (-126.4238, 85.0633) -> (-126.7296, 84.4656) centre (-98.9805, 70.6479) ccw projected
  arc A273 (-126.7296, 84.4656) -> (-128.6335, 84.6672) centre (-129.0257, 71.8732) ccw projected
  arc A274 (-128.6335, 84.6672) -> (-128.8558, 84.1869) centre (-98.9805, 70.6479) ccw projected
  arc A275 (-128.8558, 84.1869) -> (-127.4702, 82.8657) centre (-119.3545, 92.7639) ccw projected
  arc A276 (-127.4702, 82.8657) -> (-127.7281, 82.2458) centre (-98.9805, 70.6479) ccw projected
  arc A277 (-127.7281, 82.2458) -> (-129.642, 82.2974) centre (-129.0292, 69.5121) ccw projected
  arc A278 (-129.642, 82.2974) -> (-129.826, 81.8012) centre (-98.9805, 70.6479) ccw projected
  arc A279 (-129.826, 81.8012) -> (-128.341, 80.5927) centre (-121.0269, 91.0972) ccw projected
  arc A280 (-128.341, 80.5927) -> (-128.5495, 79.9545) centre (-98.9805, 70.6479) ccw projected
  arc A281 (-128.5495, 79.9545) -> (-130.4615, 79.8558) centre (-128.8474, 67.158) ccw projected
  arc A282 (-130.4615, 79.8558) -> (-130.606, 79.3467) centre (-98.9805, 70.6479) ccw projected
  arc A283 (-130.606, 79.3467) -> (-129.0307, 78.2585) centre (-122.5633, 89.3044) ccw projected
  arc A284 (-129.0307, 78.2585) -> (-129.1885, 77.6059) centre (-98.9805, 70.6479) ccw projected
  arc A285 (-129.1885, 77.6059) -> (-131.0869, 77.3575) centre (-128.4816, 64.8254) ccw projected
  arc A286 (-131.0869, 77.3575) -> (-131.191, 76.8386) centre (-98.9805, 70.6479) ccw projected
  arc A287 (-131.191, 76.8386) -> (-129.5352, 75.8773) centre (-123.9544, 87.3966) ccw projected
  arc A288 (-129.5352, 75.8773) -> (-129.6413, 75.2143) centre (-98.9805, 70.6479) ccw projected
  arc A289 (-129.6413, 75.2143) -> (-131.5144, 74.8177) centre (-127.9338, 62.5287) ccw projected
  arc A290 (-131.5144, 74.8177) -> (-131.5774, 74.2923) centre (-98.9805, 70.6479) ccw projected
  arc A291 (-131.5774, 74.2923) -> (-129.8513, 73.4639) centre (-125.1915, 85.3856) ccw projected
  arc A292 (-129.8513, 73.4639) -> (-129.9051, 72.7946) centre (-98.9805, 70.6479) ccw projected
  arc A293 (-129.9051, 72.7946) -> (-131.7412, 72.2523) centre (-127.2075, 60.2821) ccw projected
  arc A294 (-131.7412, 72.2523) -> (-131.7628, 71.7235) centre (-98.9805, 70.6479) ccw projected
  arc A295 (-131.7628, 71.7235) -> (-129.9771, 71.0331) centre (-126.267, 83.2836) ccw projected
  arc A296 (-129.9771, 71.0331) -> (-129.9782, 70.3617) centre (-98.9805, 70.6479) ccw projected
  arc A297 (-129.9782, 70.3617) -> (-131.7661, 69.677) centre (-126.3072, 58.0994) ccw projected
  arc A298 (-131.7661, 69.677) -> (-131.7462, 69.1482) centre (-98.9805, 70.6479) ccw projected
  arc A299 (-131.7462, 69.1482) -> (-129.9118, 68.6) centre (-127.1743, 81.1038) ccw projected
  arc A300 (-129.9118, 68.6) -> (-129.8602, 67.9305) centre (-98.9805, 70.6479) ccw projected
  arc A301 (-129.8602, 67.9305) -> (-131.5889, 67.1076) centre (-125.2384, 55.9941) ccw projected
  arc A302 (-131.5889, 67.1076) -> (-131.5275, 66.582) centre (-98.9805, 70.6479) ccw projected
  arc A303 (-131.5275, 66.582) -> (-129.6557, 66.1794) centre (-127.9077, 78.8595) ccw projected
  arc A304 (-129.6557, 66.1794) -> (-129.5518, 65.5161) centre (-98.9805, 70.6479) ccw projected
  arc A305 (-129.5518, 65.5161) -> (-131.2106, 64.5601) centre (-124.0077, 53.9791) ccw projected
  arc A306 (-131.2106, 64.5601) -> (-131.1082, 64.0409) centre (-98.9805, 70.6479) ccw projected
  arc A307 (-131.1082, 64.0409) -> (-129.2106, 63.7865) centre (-128.4628, 76.5646) ccw projected
  arc A308 (-129.2106, 63.7865) -> (-129.0549, 63.1334) centre (-98.9805, 70.6479) ccw projected
  arc A309 (-129.0549, 63.1334) -> (-130.6336, 62.0502) centre (-122.6228, 52.0668) ccw projected
  arc A310 (-130.6336, 62.0502) -> (-130.4907, 61.5406) centre (-98.9805, 70.6479) ccw projected
  arc A311 (-130.4907, 61.5406) -> (-128.579, 61.4358) centre (-128.8361, 74.2332) ccw projected
  arc A312 (-128.579, 61.4358) -> (-128.3726, 60.7969) centre (-98.9805, 70.6479) ccw projected
  arc A313 (-128.3726, 60.7969) -> (-129.8614, 59.5932) centre (-121.092, 50.2692) ccw projected
  arc A314 (-129.8614, 59.5932) -> (-129.6791, 59.0964) centre (-98.9805, 70.6479) ccw projected
  arc A315 (-129.6791, 59.0964) -> (-127.765, 59.1419) centre (-129.0254, 71.8797) ccw projected
  arc A316 (-127.765, 59.1419) -> (-127.5091, 58.5212) centre (-98.9805, 70.6479) ccw projected
  arc A317 (-127.5091, 58.5212) -> (-128.8989, 57.2044) centre (-119.425, 48.5971) ccw projected
  arc A318 (-128.8989, 57.2044) -> (-128.6781, 56.7234) centre (-98.9805, 70.6479) ccw projected
  arc A319 (-128.6781, 56.7234) -> (-126.7735, 56.919) centre (-129.0294, 69.5186) ccw projected
  arc A320 (-126.7735, 56.919) -> (-126.4697, 56.3203) centre (-98.9805, 70.6479) ccw projected
  circle A321 centre (-98.9805, 70.6479) radius 4 projected
  circle A322 centre (-102.0302, 78.0439) radius 1.75 projected
  circle A323 centre (-95.9308, 63.252) radius 1.75 projected
  circle A324 centre (-91.5846, 73.6976) radius 1.75 projected
  circle A325 centre (-106.3764, 67.5983) radius 1.75 projected
  circle A326 centre (-117.528, 78.4842) radius 4 projected
  circle A327 centre (-91.3824, 89.3012) radius 4 projected
  circle A328 centre (-80.4524, 62.8124) radius 4 projected
  circle A329 centre (-106.8822, 52.1244) radius 4 projected
  circle A330 centre (-106.6288, 89.1962) radius 4 projected
  circle A331 centre (-91.3243, 52.0805) radius 4 projected
  circle A332 centre (-80.4322, 78.2962) radius 4 projected
  circle A333 centre (-117.548, 62.9917) radius 4 projected
  line L0 (-98.9805, 70.6479) -> (-98.9805, 0)
  line L1 (-203.2, 0) -> (0, 0) projected
  constraints: 2 end point, 1 point on line, 1 vertical
sketch "Sketch4" plane through (0, 3.302, 0) normal (0, 1, 0) x (1, 0, 0)
  circle A0 centre (-99.0482, 22.5236) radius 4 projected
  point P0 (0, 0)
extrude "Extrusion3" cut sketch "Sketch4" against normal blind 14.2875
body "Solid1"
